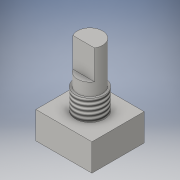
# Autodesk Inventor part: PEC11R-4215F-S0024
Saved by Autodesk Inventor 2016 (Build 200138000, 138)
## iProperties
Created: 2015-10-20
Part Number: PEC11R-4215F-S0024
Material: Generic
Document SubType Name: Modeling
Designer: jeremyhale
Density: 1 g/cm^3
Appearance: Default
Author: jeremyhale
Autodesk Inventor part; units mm, degrees
ref_plane "YZ Plane" through (0, 0, 0) normal (1, 0, 0) x (0, 1, 0)
ref_plane "XZ Plane" through (0, 0, 0) normal (0, 1, 0) x (-1, 0, 0)
ref_plane "XY Plane" through (0, 0, 0) normal (0, 0, 1) x (1, 0, 0)
sketch "Sketch1" plane through (0, 0, 0) normal (0, 1, 0) x (-1, 0, 0)
  line L0 (-6.7, 6.25) -> (6.7, 6.25)
  line L1 (6.7, 6.25) -> (6.7, -6.25)
  line L2 (6.7, -6.25) -> (-6.7, -6.25)
  line L3 (-6.7, -6.25) -> (-6.7, 6.25)
  line L4 (-6.7, 6.25) -> (6.7, -6.25) construction
  line L5 (6.7, 6.25) -> (-6.7, -6.25) construction
  point P0 (0, 0)
  dimension "d0" = 13.4
  dimension "d1" = 12.5
  constraints: 12 end point, 2 midpoint, 2 parallel, 1 horizontal, 1 perpendicular
  measures "d0" distance of L1.end L2.end
  measures "d1" distance of L0.end L1.end
extrude "Extrusion1" add sketch "Sketch1" along normal blind 6.5
sketch "Sketch2" plane through (0, 6.5, 0) normal (0, 1, 0) x (1, 0, 0)
  circle A0 centre (0, 0) radius 3.5
  dimension "d4" = 7
  constraints: 1 centre point, 1 coincident
  measures "d4" diameter of A0
extrude "Extrusion2" add sketch "Sketch2" along normal blind 5
sketch "Sketch3" plane through (0, 11.5, 0) normal (0, 1, 0) x (1, 0, 0)
  circle A0 centre (0, 0) radius 3
  dimension "d7" = 6
  constraints: 1 centre point, 1 coincident
  measures "d7" diameter of A0
extrude "Extrusion3" add sketch "Sketch3" along normal blind 10
sketch "Sketch4" plane through (0, 21.5, 0) normal (0, 1, 0) x (1, 0, 0)
  line L0 (0, -1.5) -> (2.5981, -1.5)
  circle A0 centre (0, 0) radius 3 projected
  line L1 (0, -1.5) -> (-2.5981, -1.5)
  arc A1 (-2.5981, -1.5) -> (2.5981, -1.5) centre (0, 0) ccw
  dimension "d10" = 1.5
  constraints: 4 end point, 4 point on circle, 2 horizontal, 1 centre point, 1 coincident
  measures "d10" distance from line of point (0, 0) L0
extrude "Extrusion4" cut sketch "Sketch4" against normal blind 7 contours L0 A0 L1 picked at (-1.5934, -1.6862)
thread "Thread1" size "M7x1" class "6g" standard "ISO Metric profile" full length
body "Solid1"
